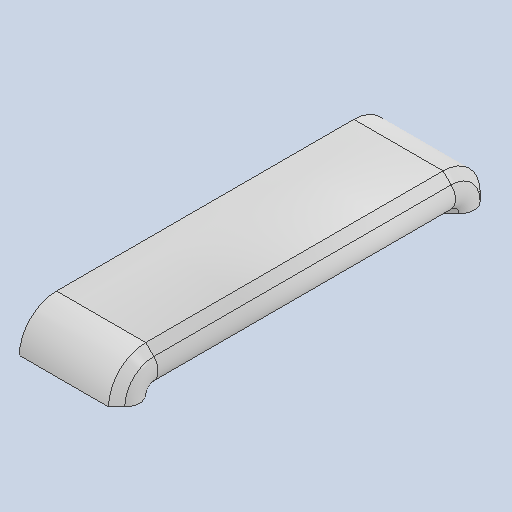
# Autodesk Inventor part: 窗頂_2
Saved by Autodesk Inventor 2024.2 (Build 282272000, 272)
## iProperties
Created: 2024-06-02
Part Number: 窗頂_2
Material: 一般
Document SubType Name: Modeling
Designer: User
Density: 1 g/cm^3
Appearance: 預設
Author: User
Autodesk Inventor part; units mm, degrees
ref_plane "YZ Plane" through (0, 0, 0) normal (1, 0, 0) x (0, 1, 0)
ref_plane "XZ Plane" through (0, 0, 0) normal (0, 1, 0) x (-1, 0, 0)
ref_plane "XY Plane" through (0, 0, 0) normal (0, 0, 1) x (1, 0, 0)
sketch "草圖1" plane through (0, 0, 0) normal (0, 0, 1) x (1, 0, 0)
  line L0 (0, 0) -> (0.6, 0)
  line L1 (0.6, 0) -> (0.6, 0.25)
  line L2 (0.6, 0.25) -> (0, 0.25)
  line L3 (0, 0.25) -> (0, 0)
  line L4 (0.6, 0.25) -> (0.725, 0.125)
  line L5 (0.725, 0.125) -> (0.6, 0)
  dimension "d0" = 0.6
  dimension "d1" = 0.25
  dimension "d2" = 45
  constraints: 12 end point, 2 parallel, 2 perpendicular, 1 horizontal
  measures "d0" distance of L0.start L0.end
  measures "d1" distance of L1.end L0.end
  measures "d2" angle of L1 L4
extrude "擠出1" add sketch "草圖1" along normal blind 2
sketch "草圖2" plane through (0, 0, 2) normal (0, 0, 1) x (1, 0, 0)
  line L0 (0, 0.25) -> (0, 0) projected
  line L1 (0, 0.25) -> (0, 0)
  line L2 (0, 0.25) -> (0, 0) projected
  line L3 (0, 0) -> (0.6, 0) projected
  line L4 (0.6, 0) -> (0.725, 0.125) projected
  line L5 (0.725, 0.125) -> (0.6, 0.25) projected
  line L6 (0.6, 0.25) -> (0, 0.25) projected
  line L7 (0.6, 0.25) -> (0.725, 0.125)
  line L8 (0, 0) -> (0.6, 0) projected
  line L9 (0.6, 0) -> (0, 0)
  line L10 (0, 0) -> (0, 0.25)
  line L11 (0.6, 0.25) -> (0, 0.25)
  constraints: 10 end point, 5 collinear
revolve "迴轉1" add sketch "草圖2" angle 90 about axis through (0, 0, 2) along (1, 0, 0)
sketch "草圖3" plane through (0, 0, 0) normal (0, 0, -1) x (-1, 0, 0)
  line L0 (-0.6, 0.25) -> (0, 0.25) projected
  line L1 (-0.725, 0.125) -> (-0.6, 0.25) projected
  line L2 (-0.6, 0.25) -> (-0.725, 0.125)
  line L3 (-0.725, 0.125) -> (-0.6, 0)
  line L4 (0, 0) -> (-0.6, 0) projected
  line L5 (-0.6, 0) -> (0, 0)
  line L6 (0, 0.25) -> (0, 0) projected
  line L7 (0, 0) -> (0, 0.25)
  line L8 (0, 0.25) -> (-0.6, 0.25)
  constraints: 10 end point, 3 perpendicular, 2 collinear
revolve "迴轉2" add sketch "草圖3" angle 90 about axis through (0, 0, 0) along (-1, 0, 0)
fillet "圓角1" radius 0.1 3 edges at (0.725, 0.0884, 2.0884) (0.725, 0.0884, -0.0884) (0.725, 0.125, 1)
